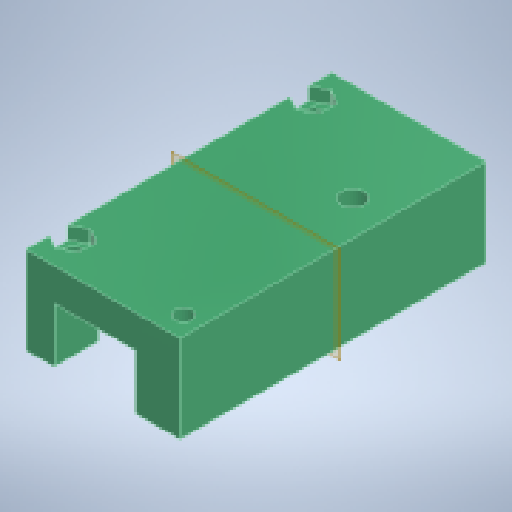
# Autodesk Inventor part: креп_центр_м2
Saved by Autodesk Inventor 2023.1 (Build 271208000, 208)
## iProperties
Created: 2025-12-23
Part Number: креп_центр_м2
Material: Полипропилен
Document SubType Name: Sheet Metal
Designer: DELL
Density: 0.899 g/cm^3
Appearance: Гладкий — темный цвет морской волны
Sheet Metal Rule: По умолчанию
Author: DELL
Autodesk Inventor part; units mm, degrees
ref_plane "YZ Plane" through (0, 0, 0) normal (1, 0, 0) x (0, 1, 0)
ref_plane "XZ Plane" through (0, 0, 0) normal (0, 1, 0) x (-1, 0, 0)
ref_plane "XY Plane" through (0, 0, 0) normal (0, 0, 1) x (1, 0, 0)
sketch "Эскиз1" plane through (0, 0, 0) normal (0, 0, 1) x (1, 0, 0)
  line L0 (0, 0) -> (-20, 0) construction
  line L1 (-20, 0) -> (-20, 10) construction
  line L2 (-20, 10) -> (0, 10) construction
  line L3 (0, 10) -> (0, 0) construction
  line L4 (-20, 0) -> (8.2, 0) construction
  line L5 (8.2, 0) -> (8.2, 16)
  line L6 (8.2, 16) -> (-20, 16)
  line L7 (-20, 16) -> (-20, 0) construction
  line L8 (-20, 16) -> (-20, 10)
  line L9 (-20, 10) -> (0, 10)
  line L10 (0, 10) -> (0, 0)
  line L11 (0, 0) -> (8.2, 0)
  point P0 (-10, 10)
  dimension "d0" = 20
  dimension "d1" = 10
  dimension "d2" = 6
  dimension "d3" = 8.2
  constraints: 24 end point, 4 parallel, 3 collinear, 3 perpendicular, 2 horizontal, 1 midpoint
  measures "d0" distance of L1.end L2.end
  measures "d1" distance of L0.end L1.end
  measures "d2" distance from line of L6 point (-10, 10)
  measures "d3" distance between parallel lines of L5 L3
extrude "Выдавливание1" add sketch "Эскиз1" along normal blind 56
sketch "Эскиз5" plane through (-20, 10, 0) normal (-1, 0, 0) x (0, 0, 1)
  line L0 (0, 0) -> (56, 0) projected
  line L1 (0, -10) -> (56, -10) projected
  line L2 (56, 0) -> (48, 0)
  line L3 (48, 0) -> (48, -10)
  line L4 (48, -10) -> (56, -10)
  line L5 (56, -10) -> (56, 0)
  line L6 (0, 0) -> (8, 0)
  line L7 (8, 0) -> (8, -10)
  line L8 (8, -10) -> (0, -10)
  line L9 (0, -10) -> (0, 0)
  point P0 (48, 0)
  point P1 (8, -10)
  point P2 (8, 0)
  dimension "d37" = 8
  dimension "d38" = 8
  constraints: 16 end point, 4 parallel, 3 point on line, 2 horizontal, 2 perpendicular
  measures "d37" distance of L4.end L3.end
  measures "d38" distance of L7.end L8.end
extrude "Выдавливание5" add sketch "Эскиз5" against normal blind 5.2 contours L0 L7 L1 L9 | L0 L5 L1 L3
sketch "Эскиз6" plane through (-20, 0, 48) normal (0, -1, 0) x (1, 0, 0)
  line L0 (0, 0) -> (0, 8) projected
  line L1 (0, 0) -> (5.2, 0) projected
  line L2 (5.2, 8) -> (5.2, 0) projected
  line L3 (0, 8) -> (5.2, 8) projected
  circle A0 centre (2.6, 2) radius 1.6
  line L4 (2.6, 2) -> (5.2, 4)
  line L5 (2.6, 2) -> (0, 4)
  line L6 (0, 0) -> (0, 8) projected
  point P0 (20, -48)
  dimension "d41" = 3.2
  dimension "d45" = 6
  constraints: 4 end point, 2 midpoint, 1 centre point, 1 equal length
  measures "d41" diameter of A0
  measures "d45" distance from line of L3 L4.start
extrude "Выдавливание6" cut sketch "Эскиз6" against normal blind 20 contours L5 L4 A0 | A0 L4 L5
sketch "Эскиз7" plane through (-20, 16, 0) normal (0, 1, 0) x (1, 0, 0)
  circle A0 centre (2.6, -50) radius 1.6 projected
  line L0 (5.35, -48.4123) -> (5.35, -51.5877)
  line L1 (5.35, -51.5877) -> (2.6, -53.1754)
  line L2 (2.6, -53.1754) -> (-0.15, -51.5877)
  line L3 (-0.15, -51.5877) -> (-0.15, -48.4123)
  line L4 (-0.15, -48.4123) -> (2.6, -46.8246)
  line L5 (2.6, -46.8246) -> (5.35, -48.4123)
  line L6 (0, 0) -> (0, -56) projected
  point P0 (20, 0)
  point P1 (0, -48.3257)
  point P2 (0, -51.6743)
  dimension "d44" = 5.5
  constraints: 12 end point, 1 coincident, 1 parallel, 13 other
  measures "d44" distance between parallel lines of L3 L0
extrude "Выдавливание7" cut sketch "Эскиз7" against normal blind 2.4 contours L0 L1 L2 L6 L4 L5
ref_plane "РабПлоскость1" through (0, 0, 28) normal (0, 0, 1) x (1, 0, 0)
mirror "Зеркальное отражение1" about plane through (0, 0, 28) normal (0, 0, 1) of "Выдавливание6", "Выдавливание7"
sketch "Эскиз8" plane through (-20, 16, 0) normal (0, 1, 0) x (1, 0, 0)
  circle A0 centre (24.8, -52) radius 1.6
  circle A1 centre (24.8, -18) radius 1.6 construction
  line L0 (24.8, -52) -> (24.8, -18)
  line L1 (28.2, 0) -> (28.2, -56) projected
  line L2 (0, -7.6743) -> (0, -48.3257) projected
  line L3 (28.2, -56) -> (0, -56) projected
  point P0 (20, 0)
  dimension "d49" = 3.2
  dimension "d50" = 3.2
  dimension "d51" = 34
  dimension "d52" = 24.8
  dimension "d53" = 4
  constraints: 2 centre point, 2 end point, 1 parallel
  measures "d49" diameter of A0
  measures "d50" diameter of A1
  measures "d51" distance of L0.start L0.end
  measures "d52" distance from line of L2 L0.end
  measures "d53" distance from line of L3 L0.start
extrude "Выдавливание8" cut sketch "Эскиз8" against normal blind 56
sketch "Эскиз9" plane through (-20, 16, 0) normal (0, 1, 0) x (1, 0, 0)
  circle A0 centre (9.8, 137.0813) radius 6 projected
  line L0 (15.8, 137.0813) -> (15.8, -29.0562) construction
  circle A1 centre (21.8, -18) radius 6 construction
  circle A2 centre (21.8, -18) radius 2.1
  point P0 (20, 0)
  dimension "d56" = 12
  dimension "d57" = 18
  dimension "d58" = 4.2
  constraints: 2 centre point, 2 end point, 2 vertical, 1 coincident, 1 horizontal alignment, 1 tangent, 1 other
  measures "d56" diameter of A1
  measures "d57" vertical distance of point (20, 0) A1.centre
  measures "d58" diameter of A2
extrude "Выдавливание9" cut sketch "Эскиз9" against normal blind 5 contours A2
equation "\"Радиус_гибки\" = Толщина"
equation "\"Ширина_просечки\" = Толщина"
equation "\"Глубина_просечки\" = 0.5 * Толщина"
equation "\"Размер_просечки\" = 4 * Толщина"
equation "\"Мин_остаток\" = 2 * Толщина"
equation "\"Радиус_перехода\" = Радиус_гибки"
equation "\"Радиус_Якоби\" = Радиус_гибки"
equation "\"Размер_зазора\" = Толщина"
equation "\"Толщина\" = 3.048"
